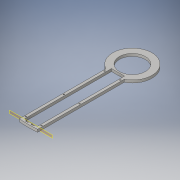
# Autodesk Inventor part: Arm Layer 2
Saved by Autodesk Inventor 2016 (Build 200138000, 138)
## iProperties
Created: 2016-04-23
Part Number: Arm Layer 2
Material: Generic
Document SubType Name: Modeling
Designer: rubenjm
Density: 1 g/cm^3
Appearance: Default
Author: rubenjm
Autodesk Inventor part; units mm, degrees
ref_plane "YZ Plane" through (0, 0, 0) normal (1, 0, 0) x (0, 1, 0)
ref_plane "XZ Plane" through (0, 0, 0) normal (0, 1, 0) x (-1, 0, 0)
sketch "Sketch2" plane through (0, 0, 0) normal (0, 1, 0) x (-1, 0, 0)
  arc A0 (44.45, 506.057) -> (-44.45, 506.057) centre (0, -1.4242) ccw construction
  arc A1 (44.45, 506.057) -> (-44.45, 506.057) centre (0, -1.4242) ccw
  line L0 (44.45, 84.2423) -> (44.45, 506.057)
  line L1 (-44.45, 506.057) -> (-44.45, 84.2423)
  circle A2 centre (0, 0) radius 57.15 construction
  circle A3 centre (0, 0) radius 63.5
  arc A4 (-44.45, 84.2423) -> (44.45, 84.2423) centre (0, 0) ccw
  line L2 (0, 0) -> (0, 508) construction
  arc A5 (31.75, 494.2843) -> (-31.75, 494.2843) centre (0, -1.4242) ccw
  line L3 (-31.75, 494.2843) -> (-31.75, 69.85)
  arc A6 (-31.75, 77.0401) -> (31.75, 77.0401) centre (0, 0) ccw construction
  line L4 (31.75, 69.85) -> (31.75, 494.2843)
  arc A7 (31.75, 62.217) -> (-31.75, 62.217) centre (0, 0) ccw construction
  line L5 (0, 69.85) -> (0, 63.5) construction
  line L6 (-31.75, 69.85) -> (31.75, 69.85)
  point P0 (-7.0927, 251.5509)
  dimension "d23" = 127
  dimension "d21" = 88.9
  dimension "d22" = 114.3
  dimension "d24" = 190.5
  dimension "d25" = 508
  dimension "d26" = 88.9
  dimension "d29" = 12.7
  dimension "d31" = 139.7
  dimension "d69" = 12.7
  dimension "d70" = 12.7
  constraints: 14 end point, 14 point on circle, 7 centre point, 4 coincident, 4 point on line, 2 parallel, 1 concentric, 1 perpendicular, 1 vertical alignment, 2 other
  measures "d21" distance of L1.start L0.end
  measures "d22" diameter of A2
  measures "d24" diameter of A4
  measures "d25" distance of L2.start L2.end
  measures "d26" distance between parallel lines of L1 L0
  measures "d29" distance between parallel lines of L0 L4
  measures "d31" diameter of A7
  measures "d69" distance between parallel lines of L1 L3
  measures "d70" radial gap between concentric circles of A1 A5
extrude "Extrusion2" add sketch "Sketch2" along normal blind 12.7
sketch "Sketch3" plane through (0, 12.7, 0) normal (0, 1, 0) x (1, 0, 0)
  arc A0 (-44.4483, -506.0602) -> (44.4517, -506.0602) centre (0.0017, 1.4211) ccw construction
  line L0 (44.4517, -506.0602) -> (44.4517, -84.2454) construction
  line L1 (-44.4483, -506.0602) -> (44.4517, -506.0602) construction
  line L2 (44.4517, -506.0602) -> (44.4517, -84.2454) construction
  line L3 (44.4517, -84.2454) -> (-44.4483, -84.2454) construction
  line L4 (-44.4483, -84.2454) -> (-44.4483, -506.0602) construction
  line L5 (-44.4483, -84.2454) -> (-44.4483, -506.0602) construction
  line L6 (-44.4483, -295.1528) -> (-38.0983, -295.1528) construction
  line L7 (-38.0983, -295.1528) -> (-38.0983, -506.0602) construction
  line L8 (-38.0983, -295.1528) -> (-38.0983, -84.2454) construction
  circle A1 centre (-38.0983, -96.9454) radius 3.175
  circle A2 centre (-38.0983, -480.6602) radius 3.175
  circle A3 centre (-38.0983, -295.1528) radius 3.175
  line L9 (0.0017, -506.0602) -> (0.0017, 1.4211) construction
  circle A4 centre (38.1017, -295.1528) radius 3.175
  line L10 (44.4517, -295.1528) -> (38.1017, -295.1528) construction
  circle A5 centre (38.1017, -96.9454) radius 3.175
  circle A6 centre (38.1017, -480.6602) radius 3.175
  line L11 (38.1017, -295.1528) -> (38.1017, -506.0602) construction
  line L12 (38.1017, -295.1528) -> (38.1017, -84.2454) construction
  line L13 (44.4517, -84.2454) -> (44.4517, -506.0602) construction
  line L14 (44.4517, -84.2454) -> (44.4517, -506.0602) construction
  point P0 (0, 0)
  dimension "d54" = 6.35
  dimension "d55" = 90
  dimension "d56" = 6.35
  dimension "d57" = 12.7
  dimension "d58" = 6.35
  dimension "d59" = 6.35
  dimension "d60" = 25.4
  constraints: 30 end point, 8 symmetric about line, 7 centre point, 5 point on line, 2 coincident, 2 horizontal, 2 midpoint, 2 parallel, 2 point on circle, 1 perpendicular, 1 vertical, 3 other
  measures "d54" distance of L6.start L6.end
  measures "d55" angle of L6 L7
  measures "d56" diameter of A1
  measures "d57" distance from line of A1.centre L3
  measures "d58" diameter of A2
  measures "d59" diameter of A3
  measures "d60" distance of L7.end A2.centre
extrude "Extrusion3" cut sketch "Sketch3" against normal blind 12.7
ref_plane "Work Plane2" through (0, 0, 494.411) normal (0, 0, 1) x (1, 0, 0)
sketch "Sketch5" plane through (0, 0, 494.411) normal (0, 0, 1) x (1, 0, 0)
  line L0 (-28.194, 25.4) -> (-28.194, 12.7) construction
  line L1 (-28.194, 25.4) -> (-15.494, 25.4) construction
  line L2 (-28.194, 12.7) -> (28.194, 12.7) construction
  line L3 (0, 12.7) -> (-28.194, 12.7) construction
  circle A0 centre (-14.097, 12.7) radius 6.35
  line L4 (0, 12.7) -> (0, 25.4) construction
  circle A1 centre (14.097, 12.7) radius 6.35
  line L5 (95.25, 12.7) -> (-95.25, 12.7) construction
  line L6 (95.25, 12.7) -> (-95.25, 12.7) construction
  line L7 (0, 12.7) -> (0, 0) construction
  line L8 (95.25, 0) -> (-95.25, 0) construction
  point P0 (44.45, 12.7)
  point P1 (44.45, 0)
  point P2 (-44.45, 0)
  dimension "d62" = 12.7
  dimension "d63" = 90
  dimension "d64" = 56.388
  dimension "d65" = 90
  dimension "d66" = 12.7
  constraints: 14 end point, 4 midpoint, 2 centre point, 2 horizontal, 2 perpendicular, 1 symmetric about line, 1 vertical, 1 other
  measures "d62" distance of L0.start L0.end
  measures "d63" angle of L0 L1
  measures "d64" distance of L0.end L2.end
  measures "d65" angle of L2 L0
  measures "d66" diameter of A0
extrude "Extrusion5" cut sketch "Sketch5" along normal blind 6.35
equation "\"d26\" = d21"
body "Solid2"
